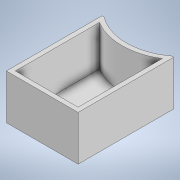
# Autodesk Inventor part: ProkladkaA
Saved by Autodesk Inventor 2022 (Build 260153000, 153)
## iProperties
Created: 2023-08-16
Part Number: ProkladkaA
Material: Generic
Document SubType Name: Modeling
Designer: Kippi
Density: 1 g/cm^3
Appearance: Default
Author: Kippi
Autodesk Inventor part; units mm, degrees
ref_plane "YZ Plane" through (0, 0, 0) normal (1, 0, 0) x (0, 1, 0)
ref_plane "XZ Plane" through (0, 0, 0) normal (0, 1, 0) x (-1, 0, 0)
ref_plane "XY Plane" through (0, 0, 0) normal (0, 0, 1) x (1, 0, 0)
sketch "Sketch1" plane through (0, 0, 0) normal (0, 1, 0) x (-1, 0, 0)
  line L0 (56.8, 106.5) -> (-103.2, 106.5)
  line L1 (-103.2, 106.5) -> (-103.2, -106.5)
  line L2 (-103.2, -106.5) -> (56.8, -106.5)
  line L3 (56.8, -106.5) -> (56.8, 106.5)
  circle A0 centre (-23.2, -206.5) radius 125
  point P0 (0, 0)
  point P1 (-98.2, -106.5)
  point P2 (51.8, -106.5)
  dimension "d0" = 213
  dimension "d1" = 160
  dimension "d5" = 250
  dimension "d6" = 100
  constraints: 8 end point, 2 parallel, 1 centre point, 1 horizontal, 1 perpendicular
  measures "d0" distance of L2.end L0.start
  measures "d1" distance of L0.start L0.end
  measures "d5" diameter of A0
  measures "d6" distance from line of L2 A0.centre
extrude "Extrusion1" add sketch "Sketch1" along normal blind 100 contours L3 L2 A0 L1 L0
shell "Shell1" thickness 10 removed faces 1 at (25.6361, 100, 43.7621)
body "Solid1"
